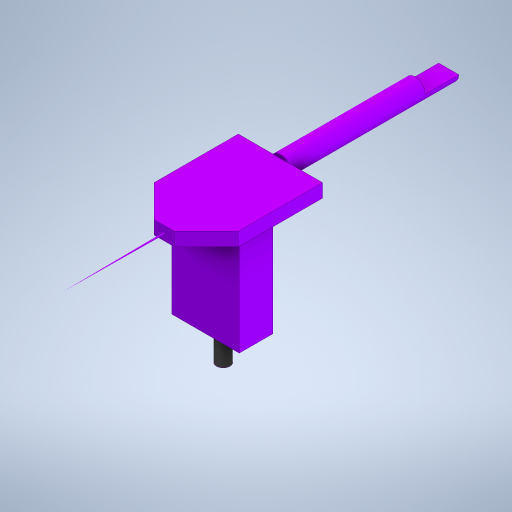
# Autodesk Inventor part: electrode
Saved by Autodesk Inventor 2024 (Build 280153000, 153)
## iProperties
Created: 2021-02-23
Part Number: electrode
Material: Generic
Document SubType Name: Modeling
Designer: dsdan
Density: 1 g/cm^3
Appearance: Default
Author: dsdan
Autodesk Inventor part; units mm, degrees
ref_plane "YZ Plane" through (0, 0, 0) normal (1, 0, 0) x (0, 1, 0)
ref_plane "XZ Plane" through (0, 0, 0) normal (0, 1, 0) x (-1, 0, 0)
ref_plane "XY Plane" through (0, 0, 0) normal (0, 0, 1) x (1, 0, 0)
sketch "Sketch1" plane through (0, 0, 0) normal (0, 0, 1) x (1, 0, 0)
  circle A0 centre (0, 0) radius 3
  dimension "d0" = 6
  constraints: 1 centre point, 1 coincident
  measures "d0" diameter of A0
extrude "Extrusion1" add sketch "Sketch1" along normal blind 50
sketch "Sketch2" plane through (0, 0, 0) normal (0, 1, 0) x (-1, 0, 0)
  line L0 (-12.5, 75) -> (-12.5, 50)
  line L1 (-12.5, 50) -> (12.5, 50)
  line L2 (12.5, 50) -> (12.5, 75)
  line L3 (12.5, 75) -> (-12.5, 75)
  line L4 (-12.5, 75) -> (12.5, 50) construction
  line L5 (-12.5, 50) -> (12.5, 75) construction
  line L6 (3, 50) -> (-3, 50) projected
  line L7 (3, 50) -> (-3, 50) projected
  line L8 (3, 0) -> (-3, 0) projected
  line L9 (3, 0) -> (-3, 0) projected
  line L10 (-3, 0) -> (3, 50)
  line L11 (3, 0) -> (-3, 50)
  line L12 (12.5, 75) -> (3, 84.5)
  line L13 (3, 84.5) -> (3, 84.5)
  line L14 (3, 84.5) -> (-3, 84.5)
  line L15 (-3, 84.5) -> (-3, 84.5)
  line L16 (-3, 84.5) -> (-12.5, 75)
  line L17 (0.25, 84.5) -> (0, 114.5)
  line L18 (0, 114.5) -> (-0.25, 84.5)
  line L19 (0, 114.5) -> (0, 84.5)
  point P0 (0, 0)
  point P1 (0, 62.5)
  point P2 (0, 50)
  point P3 (0, 25)
  point P4 (0, 62.5)
  dimension "d3" = 25
  dimension "d4" = 25
  dimension "d5" = 6
  dimension "d6" = 0
  dimension "d11" = 30
  dimension "d14" = 0.5
  dimension "d15" = 0.25
  constraints: 32 end point, 7 midpoint, 5 perpendicular, 2 parallel, 2 point on line, 2 vertical, 2 vertical alignment, 1 collinear, 1 horizontal alignment
  measures "d3" distance of L0.start L0.end
  measures "d4" distance of L2.end L0.start
  measures "d5" distance between parallel lines of L15 L13
  measures "d6" distance of L12.end L13.end
  measures "d11" vertical distance of L17.end L18.end
  measures "d14" distance of L18.end L17.start
  measures "d15" distance of L19.end L17.start
extrude "Extrusion2" add sketch "Sketch2" along normal mid plane 4 contours L3 L2 L1 L0 | L16 L14 L12 L3
sketch "Sketch3" plane through (0, -2, 0) normal (0, -1, 0) x (1, 0, 0)
  line L0 (-10, 72.2148) -> (-10, 62.2148)
  line L1 (-10, 62.2148) -> (10, 62.2148)
  line L2 (10, 62.2148) -> (10, 72.2148)
  line L3 (10, 72.2148) -> (-10, 72.2148)
  line L4 (-10, 72.2148) -> (10, 62.2148) construction
  line L5 (-10, 62.2148) -> (10, 72.2148) construction
  point P0 (0, 0)
  point P1 (0, 67.2148)
  dimension "d18" = 10
  dimension "d24" = 20
  constraints: 12 end point, 2 midpoint, 2 parallel, 1 perpendicular
  measures "d18" distance of L1.end L2.end
  measures "d24" distance of L0.end L1.end
extrude "Extrusion3" add sketch "Sketch3" along normal blind 30
revolve "Revolution1" add sketch "Sketch2" angle 360 about axis through (0, 0, 114.5) along (0, 0, -1) contours L14 L19 L17
sketch "Sketch5" plane through (0, 0, 0) normal (0, 0, -1) x (-1, 0, 0)
  arc A0 (-2.2361, 2) -> (-2.2361, -2) centre (0, 0) ccw projected
  line L0 (-3, 0) -> (3.9396, 0)
  line L1 (3.9396, 0) -> (3.9396, 5.4672)
  line L2 (3.9396, 5.4672) -> (-3, 5.4672)
  line L3 (-3, 5.4672) -> (-3, 0)
  constraints: 8 end point, 2 parallel, 1 horizontal, 1 perpendicular, 1 point on circle
extrude "Extrusion4" cut sketch "Sketch5" against normal blind 10
sketch "Sketch6" plane through (0, -32, 0) normal (0, -1, 0) x (1, 0, 0)
  circle A0 centre (0, 66.9819) radius 2
  point P0 (0, 0)
  dimension "d25" = 4
  constraints: 1 centre point
  measures "d25" diameter of A0
extrude "Extrusion5" add sketch "Sketch6" along normal blind 10
equation "\"d15\" = 0.5 * d14"
body "Solid1"
